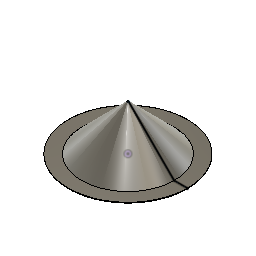
stage assembly v116 (Autodesk Fusion 360 archive; units mm, degrees)
design "electrode v2"
Autodesk Fusion 360 part; units mm, degrees
sketch "Sketch1" plane through (0, 0, 0) normal (0, 0, 1) x (1, 0, 0)
  line L0 (0.0652, 3.4348) -> (3.5, 0)
  line L1 (3.5, 0) -> (4.5, 0)
  line L2 (0.0298, 3.3994) -> (3.4793, -0.05)
  line L3 (3.4793, -0.05) -> (4.5, -0.05)
  line L4 (0.0652, 3.4348) -> (0.0298, 3.3994)
  line L5 (4.5, -0.05) -> (4.5, 0)
  dimension "d1" = 3.5
  dimension "d2" = 1
  dimension "d3" = 45
  dimension "d4" = 0.05
  constraint horizontal L1
  constraint horizontal origin L0.end
  constraint perpendicular L1 L5
  measures "d1" distance of origin L0.end
  measures "d2" distance of L0.end L1.end
  measures "d3" angle of L0 L1
revolve "Revolve1" add sketch "Sketch1" angle 360 about axis through (0, 1.75, 0) along (0, 1, 0)

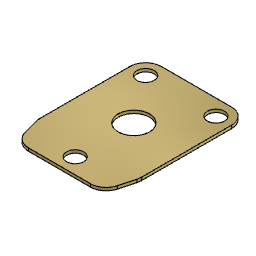
design "smb electrode top ground"
Autodesk Fusion 360 part; units mm, degrees
sketch "Sketch1" plane through (0, 0, 0) normal (0, 1, 0) x (1, 0, 0)
  circle A0 centre (-4.5, 13.5) radius 1.1
  circle A1 centre (4.5, 13.5) radius 1.1
  line L0 (0, -20) -> (0, -2.5) construction
  circle A2 centre (0, 0) radius 1.1
  circle A3 centre (0, 7.5) radius 2
  line L1 (-6.5, -2) -> (6.5, -2)
  line L2 (6.5, -2) -> (6.5, 15.5)
  line L3 (-6.5, -2) -> (-6.5, 15.5)
  line L4 (6.5, 15.5) -> (-6.5, 15.5)
  line L5 (-5.5, -2) -> (-6.5, 1.7321)
  line L6 (5.5, -2) -> (6.5, 1.7321)
  dimension "d1" = 2.2
  dimension "d2" = 2.2
  dimension "d3" = 9
  dimension "d4" = 13.5
  dimension "d5" = 2.2
  dimension "d6" = 7.5
  dimension "d7" = 4
  dimension "d8" = 13
  dimension "d9" = 2
  dimension "d10" = 2
  dimension "d15" = 30
  dimension "d16" = 11
  constraint horizontal A0.centre A1.centre
  constraint symmetric A0.centre A1.centre L0
  constraint coincident A2.centre origin
  constraint vertical A2.centre A3.centre
  constraint horizontal L1
  constraint perpendicular L1 L2
  constraint perpendicular L1 L3
  constraint perpendicular L2 L4
  constraint coincident L1 L5.start
  constraint coincident L3 L5.end
  constraint coincident L1 L6.start
  constraint coincident L2 L6.end
  constraint symmetric L0 L5 L6
  measures "d1" diameter of A0
  measures "d2" diameter of A1
  measures "d3" horizontal distance of A0.centre A1.centre
  measures "d4" vertical distance of A2.centre A1.centre
  measures "d5" diameter of A2
  measures "d6" distance of A2.centre A3.centre
  measures "d7" diameter of A3
  measures "d8" distance of L1.start L1.end
  measures "d9" distance of A2.centre L1
  measures "d10" distance of A1.centre L4
  measures "d15" angle of L5 L6
  measures "d16" distance of L5.start L6.start
extrude "Extrude1" add sketch "Sketch1" along normal blind 0.38 contours L1 L2 L3 L4 L5 L6
fillet "Fillet1" radius 2 6 edges at (-6.5, 0.19, -15.5) (6.5, 0.19, -15.5) (-5.5, 0.19, 2) (-6.5, 0.19, -1.7321) (5.5, 0.19, 2) (6.5, 0.19, -1.7321)

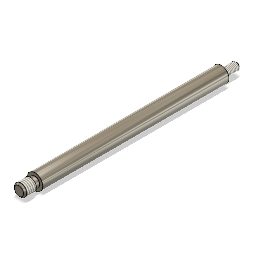
design "stage standoffs"
Autodesk Fusion 360 part; units mm, degrees
sketch "Sketch1" plane through (0, 0, 0) normal (1, 0, 0) x (0, 0, -1)
  line L0 (0, 0) -> (-137, 0)
  line L1 (-137, 0) -> (-137, 4)
  line L2 (-137, 4) -> (-127, 4)
  line L3 (-127, 4) -> (-127, 5)
  line L4 (-127, 5) -> (-10, 5)
  line L5 (-10, 5) -> (-10, 2.5)
  line L6 (-10, 2.5) -> (0, 2.5)
  line L7 (0, 2.5) -> (0, 0)
  line L8 (-127, 4) -> (-127, 3)
  line L9 (-127, 3) -> (-130, 3)
  line L10 (-130, 3) -> (-130, 4)
  dimension "d1" = 117
  dimension "d2" = 4
  dimension "d3" = 10
  dimension "d4" = 10
  dimension "d5" = 2.5
  dimension "d6" = 5
  dimension "d7" = 3
  dimension "d8" = 1
  measures "d2" distance of L0 L2
  measures "d3" distance of L1 L3
  measures "d5" distance of L0 L6
  measures "d6" distance of L0 L4
  measures "d8" distance of L2 L9
revolve "Revolve1" add sketch "Sketch1" angle 360 about axis through (0, 0, 0) along (0, 0, 1) contours L0 L1 L2 L3 L4 L5 L6 L7 L8 L9 L10
thread "Thread1" "ISO Metric profile 8.0 M8x1.25 6g" major diameter 7.866 minor diameter 6.4455 pitch 1.25 angle 60 resizes the face on face at (0.3983, 3.9801, 132.3333)
thread "Thread2" "ISO Metric profile 5.0 M5x0.8 6g" major diameter 4.901 minor diameter 3.9895 pitch 0.8 angle 60 resizes the face on face at (-0.2489, 2.4876, 6.6667)
chamfer "Chamfer1" distance 1 angle 45 2 edges at (-1.4222, -3.6668, 137) (-0.8861, -2.2847, 0)

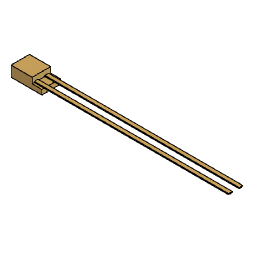
design "Lakeshore DT 670 SD Omega CY 670 SD"
Autodesk Fusion 360 part; units mm, degrees
sketch "Sketch1" plane through (0, 0, 0) normal (0, 0, 1) x (1, 0, 0)
  line L0 (0, 0) -> (3.175, 0)
  line L1 (3.175, 0) -> (3.175, 0.5)
  line L2 (3.175, 0.5) -> (2.175, 0.5)
  line L3 (2.175, 0.5) -> (2.175, 1.08)
  line L4 (2.175, 1.08) -> (0, 1.08)
  line L5 (0, 1.08) -> (0, 0)
  dimension "d1" = 1.08
  dimension "d2" = 3.175
  dimension "d3" = 1
  dimension "d4" = 0.5
  constraint coincident L0.start L5.end
  constraint horizontal L0
  constraint perpendicular L0 L1
  constraint perpendicular L1 L2
  constraint perpendicular L0 L3
  constraint perpendicular L3 L4
  constraint perpendicular L0 L5
  measures "d1" distance of L4.end L0.start
  measures "d2" distance of L0.start L0.end
  measures "d3" distance of L1.end L2.end
  measures "d4" distance of L0.end L1.end
extrude "Extrude1" add sketch "Sketch1" along normal blind 1.905
sketch "Sketch2" plane through (0, 0.5, 0) normal (0, 1, 0) x (-1, 0, 0)
  line L0 (-3.175, 0) -> (-2.175, 0)
  line L1 (-2.175, 0) -> (-2.175, 1.905)
  line L2 (-2.175, 1.905) -> (-3.175, 1.905)
  line L3 (-3.175, 1.905) -> (-3.175, 0)
  line L4 (-2.175, 0.2225) -> (-22.175, 0.2225)
  line L5 (-22.175, 0.2225) -> (-22.175, 0.6035)
  line L6 (-22.175, 0.6035) -> (-2.175, 0.6035)
  line L7 (-2.175, 0.6035) -> (-2.175, 0.2225)
  line L8 (-3.175, 0.9525) -> (0, 0.9525) construction
  line L9 (-2.175, 1.6825) -> (-22.175, 1.6825)
  line L10 (-22.175, 1.3015) -> (-2.175, 1.3015)
  line L11 (-22.175, 1.6825) -> (-22.175, 1.3015)
  line L12 (-2.175, 1.3015) -> (-2.175, 1.6825)
  dimension "d7" = 0.381
  dimension "d8" = 19
  dimension "d9" = 0.698
  constraint horizontal L4
  constraint vertical L5
  constraint horizontal L6
  constraint vertical L7
  constraint collinear L1 L7
  constraint midpoint L3 L8.start
  constraint perpendicular L3 L8
  constraint symmetric L4.start L8 L9.start
  constraint symmetric L4.end L8 L9.end
  constraint symmetric L5.end L8 L10.start
  constraint symmetric L6.end L8 L10.end
  measures "d7" distance of L4.end L5.end
  measures "d8" distance of L3 L5
  measures "d9" distance of L6 L10
extrude "Extrude2" add sketch "Sketch2" along normal blind 0.102 contours L3 L4 L5 L6 | L1 L3 L4 L6 L7 | L3 L9 L10 L11 | L1 L3 L9 L10 L12

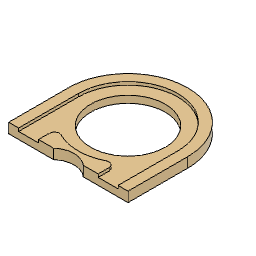
design "smb electrode insulators"
Autodesk Fusion 360 part; units mm, degrees
sketch "Sketch1" plane through (0, 0, 0) normal (0, 1, 0) x (1, 0, 0)
  line L0 (0, 0) -> (12, 0)
  line L1 (12, 0) -> (12, -12)
  line L2 (12, -12) -> (0, -12)
  line L3 (0, -12) -> (0, 0)
  circle A0 centre (6, -6) radius 3.75
  line L4 (6, 0) -> (6, -12) construction
  circle A1 centre (6, -6) radius 5
  line L5 (2, -12) -> (2, -9) construction
  line L6 (1, -12) -> (1, -6)
  line L7 (3, -10) -> (3, -12)
  arc A2 (7.5, -12) -> (4.5, -12) centre (6, -13.7) ccw
  dimension "d1" = 12
  dimension "d2" = 12
  dimension "d3" = 7.5
  dimension "d4" = 10
  dimension "d5" = 4
  dimension "d6" = 2
  dimension "d16" = 3
  dimension "d17" = 1.7
  constraint horizontal L0
  constraint vertical L1
  constraint horizontal L2
  constraint vertical L3
  constraint coincident L0.start L3.end
  constraint midpoint L0 L4.start
  constraint midpoint L2 L4.end
  constraint midpoint A0.centre L4
  constraint concentric A0 A1
  constraint coincident L2 L5.start
  constraint perpendicular L2 L5
  constraint coincident L2 L6.start
  constraint coincident A1 L6.end
  constraint perpendicular L2 L6
  constraint coincident A1 L7.start
  constraint coincident L2 L7.end
  constraint perpendicular L2 L7
  constraint coincident A1 L5.end
  constraint coincident L2 A2.start
  constraint coincident L2 A2.end
  constraint coincident L4 A2.centre
  measures "d1" distance of L0.start L2.end
  measures "d2" distance of L1.end L2.end
  measures "d3" diameter of A0
  measures "d4" diameter of A1
  measures "d5" distance of L4.end L5
  measures "d6" distance of L6 L7
  measures "d16" distance of A2.end A2.start
  measures "d17" distance of L2 A2.centre
extrude "Extrude1" add sketch "Sketch1" against normal blind 1 contours L0 L1 L2 L3 A1 L6 L7 A2 | L2 A1 L6 L7 | A1
extrude "Extrude2" cut sketch "Sketch1" against normal blind 0.3 contours A1
extrude "Extrude3" cut sketch "Sketch1" against normal blind 0.3 contours L2 A1 L6 L7
ref_plane "WorkPlane1" through (6, -0.5, 6) normal (1, 0, 0) x (0, 0, 1)
mirror "Mirror1" about plane through (6, -0.5, 6) normal (1, 0, 0) of "Extrude3"
fillet "Fillet1" radius 6 2 edges at (0, -0.5, 0) (12, -0.5, 0)
fillet "Fillet2" radius 0.5 2 edges at (3, -0.15, 10) (9, -0.15, 10)
equation "d3 = ( 3.75 * 2 ) * 1 mm"

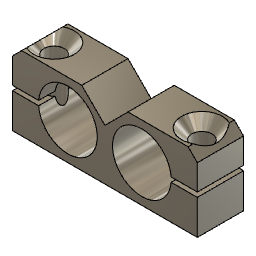
design "SMB plug holder"
Autodesk Fusion 360 part; units mm, degrees
sketch "Sketch1" plane through (0, 0, 0) normal (0, 0, 1) x (1, 0, 0)
  line L0 (0, 0) -> (20, 0)
  line L1 (20, 0) -> (20, 8)
  line L2 (20, 8) -> (0, 8)
  line L3 (0, 8) -> (0, 0)
  circle A0 centre (6, 4) radius 3.175
  circle A1 centre (14, 4) radius 3.175
  line L4 (10, 0) -> (10, 8) construction
  line L5 (7.5, 8) -> (10, 5.5)
  line L6 (10, 5.5) -> (12.5, 8)
  dimension "d1" = 6.35
  dimension "d2" = 6.35
  dimension "d3" = 8
  dimension "d4" = 4
  dimension "d5" = 20
  dimension "d6" = 8
  dimension "d9" = 2.5
  constraint horizontal L0
  constraint vertical L1
  constraint horizontal L2
  constraint vertical L3
  constraint coincident L0.start L3.end
  constraint horizontal A0.centre A1.centre
  constraint midpoint L0 L4.start
  constraint midpoint L2 L4.end
  constraint symmetric A0.centre A1.centre L4
  constraint coincident L2 L5.start
  constraint coincident L4 L5.end
  constraint coincident L2 L6.end
  constraint perpendicular L5 L6
  constraint symmetric L4 L5 L6
  measures "d1" diameter of A0
  measures "d2" diameter of A1
  measures "d3" distance of A0.centre A1.centre
  measures "d4" distance of L0 A0.centre
  measures "d5" distance of L0.start L0.end
  measures "d6" distance of L0 L2
  measures "d9" distance of L2 L5.end
extrude "Extrude1" add sketch "Sketch1" against normal blind 5 contours L0 L1 L2 L3 L5 L6
sketch "Sketch2" plane through (0, 8, 0) normal (0, 1, 0) x (-1, 0, 0)
  line L0 (-12.5, 0) -> (-20, 0)
  line L1 (-20, 0) -> (-20, -5)
  line L2 (-20, -5) -> (-12.5, -5)
  line L3 (-12.5, -5) -> (-12.5, 0)
  line L4 (0, 0) -> (0, -5)
  line L5 (-20, 0) -> (-20, -5)
  line L6 (-20, -2.5) -> (0, -2.5) construction
  line L7 (-10, 0) -> (-10, -5)
  point P0 (-2, -2.5)
  point P1 (-18, -2.5)
  dimension "d10" = 2
  dimension "d19" = 16
  constraint midpoint L1 L6.start
  constraint midpoint L4 L6.end
  constraint coincident L6 P0
  constraint coincident L6 P1
  constraint symmetric P0 P1 L7
  measures "d10" distance of L4 P0
  measures "d19" distance of P0 P1
chamfer "Chamfer1" distance 1 angle 45 2 edges at (20, 8, -2.5) (0, 8, -2.5)
hole "Hole1" at (2, 8, -2.5) at (18, 8, -2.5) direction (0, -1, 0) diameter 2.2 depth 10 tip angle 118 countersink diameter 4.4 countersink angle 90
ref_plane "WorkPlane1" through (16.25, 4, -2.5) normal (0, 1, 0) x (1, 0, 0)
sketch "Sketch3" plane through (16.25, 4, -3.5) normal (0, 1, 0) x (1, 0, 0)
  line L0 (0, 6) -> (6.8751, 6)
  line L1 (6.8751, 6) -> (6.8751, -6.5674)
  line L2 (6.8751, -6.5674) -> (0, -6.5674)
  line L3 (0, -6.5674) -> (0, 6)
  line L4 (-17, 6) -> (-11.0861, 6)
  line L5 (-11.0861, 6) -> (-11.0861, -6.5674)
  line L6 (-11.0861, -6.5674) -> (-17, -6.5674)
  line L7 (-17, -6.5674) -> (-17, 6)
  constraint horizontal L0
  constraint vertical L1
  constraint horizontal L2
  constraint vertical L3
  constraint horizontal L4
  constraint vertical L5
  constraint horizontal L6
  constraint vertical L7
extrude "Extrude2" cut sketch "Sketch3" along normal mid plane 0.5

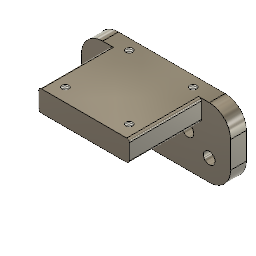
design "EX-0009723-000-XYZ-SLC-1730 z connector"
Autodesk Fusion 360 part; units mm, degrees
sketch "Sketch2" plane through (0, 0, 0) normal (0, 0, 1) x (1, 0, 0)
  arc A0 (18.5, 20) -> (18, 20.5) centre (18, 20) ccw
  line L0 (18.5, 20) -> (18.5, 8.6168)
  arc A1 (18.5, 8.6168) -> (21.6842, 3.6281) centre (24, 8.6168) ccw
  arc A2 (20, -4) -> (21.6842, 3.6281) centre (20, 0) ccw
  line L1 (20, -4) -> (0, -4)
  arc A3 (-1.6842, 3.6281) -> (0, -4) centre (0, 0) ccw
  arc A4 (-1.6842, 3.6281) -> (1.5, 8.6168) centre (-4, 8.6168) ccw
  line L2 (1.5, 8.6168) -> (1.5, 20)
  arc A5 (2, 20.5) -> (1.5, 20) centre (2, 20) ccw
  line L3 (2, 20.5) -> (18, 20.5)
  circle A6 centre (20, 0) radius 1.1
  circle A7 centre (0, 0) radius 1.1
  line L4 (24, 9) -> (-4, 9)
  line L5 (-4, 0) -> (-4, 9)
  line L6 (24, 0) -> (24, 9)
  line L7 (1.5, 9) -> (1.5, 5)
  line L8 (1.5, 5) -> (18.5, 5)
  line L9 (18.5, 5) -> (18.5, 9)
  line L10 (10, -4) -> (10, 20.5) construction
  point P0 (4, 2.5)
  point P1 (16, 2.5)
  dimension "d2" = 9
  dimension "d6" = 4
  dimension "d20" = 12
  dimension "d21" = 2.5
  constraint horizontal L4
  constraint coincident A3 L5.start
  constraint coincident A2 L6.start
  constraint tangent A2 L6
  constraint tangent A3 L5
  constraint vertical L6
  constraint vertical L5
  constraint coincident L4 L7.start
  constraint coincident L2 L7.start
  constraint perpendicular L4 L7
  constraint perpendicular L0 L8
  constraint coincident L4 L9.end
  constraint coincident L0 L9.end
  constraint perpendicular L4 L9
  constraint midpoint L1 L10.start
  constraint midpoint L3 L10.end
  constraint horizontal P0 P1
  constraint symmetric L10 P0 P1
  measures "d2" distance of A3.centre L4
  measures "d6" distance of L4 L8
  measures "d20" distance of P0 P1
  measures "d21" distance of L8 P1
ref_plane "WorkPlane1" through (0, 9, 0) normal (0, 1, 0) x (0, 0, 1)
sketch "Sketch3" plane through (0, 9, 0) normal (0, 1, 0) x (1, 0, 0)
  circle A0 centre (4, -13.5) radius 0.625
  circle A1 centre (4, -13.5) radius 0.625
  circle A2 centre (16, -13.5) radius 0.625
  circle A3 centre (16, -13.5) radius 0.625
  circle A4 centre (16, -1.5) radius 0.625
  circle A5 centre (16, -1.5) radius 0.625
  circle A6 centre (4, -1.5) radius 0.625
  circle A7 centre (4, -1.5) radius 0.625
  dimension "d4" = 12
  dimension "d5" = 12
  measures "d4" distance of A2.centre A4.centre
  measures "d5" distance of A0.centre A2.centre
extrude "Extrude1" add sketch "Sketch2" along normal blind 2.5 and the other way blind 0.5 contours L0 A1 A2 L4 L6 L9 | L0 L2 L4 L7 L8 L9 | A1 A2 L1 A3 A4 L7 L8 L9 | A3 A4 L2 L4 L5 L7
extrude "Extrude2" add sketch "Sketch2" along normal blind 16 contours L0 L2 L4 L7 L8 L9
hole "Hole1" at (4, 9, 13.5) at (16, 9, 13.5) at (16, 9, 1.5) at (4, 9, 1.5) direction (0, -1, 0) diameter 1.271 depth 6.5 tip angle 118
thread "Thread1" "ISO Metric profile 1.6 M1.6x0.35 6H"
fillet "Fillet1" radius 4 2 edges at (24, 9, 1) (-4, 9, 1)
fillet "Fillet1" radius 0.5 4 edges at (18.5, 9, 9.25) (1.5, 9, 9.25) (18.5, 5, 9.25) (1.5, 5, 9.25)
hole "Hole2" at (16, 2.5, 0) at (4, 2.5, 0) direction (0, 0, 1) diameter 2.2 depth 11 tip angle 118
hole "Hole3" at (16, 2.5, 0) at (4, 2.5, 0) direction (0, 0, -1) diameter 2.2 depth 11 tip angle 118

design "base plate"
Autodesk Fusion 360 part; units mm, degrees
sketch "Sketch1" plane through (0, 0, 0) normal (0, 1, 0) x (1, 0, 0)
  circle A0 centre (0, 0) radius 20
  line L0 (1.75, 0) -> (22.5, 0) construction
  line L1 (0, -20) -> (0, -2.5) construction
  line L2 (-35, 91) -> (35, 91)
  line L3 (35, 91) -> (35, -35)
  line L4 (35, -35) -> (-35, -35)
  line L5 (-35, -35) -> (-35, 91)
  line L6 (-8.55, 91) -> (-8.55, 25)
  line L7 (-8.55, 25) -> (8.55, 25)
  line L8 (8.55, 25) -> (8.55, 91)
  line L9 (-12.5, -25) -> (12.5, -25) construction
  circle A1 centre (-12.5, -25) radius 5
  circle A2 centre (12.5, -25) radius 5
  line L10 (-7.7, 86) -> (-7.7, 35)
  arc A3 (-7.7, 35) -> (-5.7, 35) centre (-6.7, 35) ccw
  line L11 (-5.7, 35) -> (-5.7, 86)
  arc A4 (-5.7, 86) -> (-7.7, 86) centre (-6.7, 86) ccw
  line L12 (-6.7, 86) -> (-6.7, 35) construction
  line L13 (-33, 91) -> (-33, 41)
  arc A5 (-33, 41) -> (-23, 41) centre (-28, 41) ccw
  line L14 (-23, 41) -> (-23, 91)
  line L15 (-33, 10) -> (-33, -10)
  arc A6 (-33, -10) -> (-20.592, -7.744) centre (-26.5909, -10) ccw
  arc A7 (-20.592, 7.744) -> (-33, 10) centre (-26.5909, 10) ccw
  line L16 (-26.5909, 10) -> (-26.5909, -10) construction
  line L17 (-25, -25) -> (-25, 25) construction
  line L18 (-25, 0) -> (-26.5909, 0) construction
  arc A8 (-20.592, 7.744) -> (-20.592, -7.744) centre (0, 0) ccw
  point P0 (25, 0)
  point P1 (0, -25)
  point P2 (-6.7, 66)
  point P3 (-6.7, 40)
  point P4 (6.7, 40)
  point P5 (6.7, 66)
  point P6 (-12.5, -25)
  point P7 (12.5, -25)
  point P8 (-25, 25)
  point P9 (25, 25)
  point P10 (25, -25)
  point P11 (-25, -25)
  dimension "d1" = 40
  dimension "d4" = 26
  dimension "d5" = 13.4
  dimension "d6" = 40
  dimension "d7" = 70
  dimension "d8" = 35
  dimension "d10" = 17.1
  dimension "d14" = 25
  dimension "d15" = 25
  dimension "d28" = 10
  dimension "d29" = 10
  dimension "d32" = 50
  dimension "d33" = 50
  dimension "d63" = 2
  dimension "d64" = 5
  dimension "d65" = 10
  dimension "d66" = 20
  dimension "d67" = 5
  dimension "d71" = 2
  dimension "d72" = 10
  dimension "d73" = 50
  dimension "d79" = 20
  dimension "d80" = 2
  constraint coincident A0.centre A8.centre
  constraint coincident P0 L0
  constraint horizontal P3 P4
  constraint vertical P4 P5
  constraint horizontal P2 P5
  constraint vertical P2 P3
  constraint symmetric L1 P3 P4
  constraint horizontal L2
  constraint vertical L3
  constraint horizontal L4
  constraint vertical L5
  constraint symmetric L1 L3 L5
  constraint coincident L2 L6.start
  constraint perpendicular L2 L6
  constraint perpendicular L6 L7
  constraint coincident L2 L8.end
  constraint perpendicular L2 L8
  constraint coincident L9 P6
  constraint coincident L9 P7
  constraint symmetric L1 P6 P7
  constraint coincident P7 L9.end
  constraint coincident P6 L9.start
  constraint horizontal P10 P11
  constraint vertical P8 P11
  constraint horizontal P8 P9
  constraint vertical P9 P10
  constraint symmetric L0 P9 P10
  constraint symmetric L1 P10 P11
  constraint tangent L10 A3
  constraint tangent A3 L11
  constraint parallel L10 L11
  constraint tangent L11 A4
  constraint tangent L10 A4
  constraint parallel L6 L12
  constraint coincident P3 L12
  constraint coincident L2 L13.start
  constraint perpendicular L2 L13
  constraint tangent L13 A5
  constraint coincident L2 L14.end
  constraint perpendicular L2 L14
  constraint tangent A5 L14
  constraint tangent L15 A6
  constraint tangent L15 A7
  constraint vertical L16
  constraint coincident P11 L17.start
  constraint coincident P8 L17.end
  constraint midpoint L17 L18.start
  constraint midpoint L16 L18.end
  constraint horizontal L18
  constraint collinear L13 L15
  constraint tangent A6 A8
  measures "d1" diameter of A0
  measures "d4" vertical distance of P4 P5
  measures "d5" horizontal distance of P2 P5
  measures "d6" distance of L0 P4
  measures "d7" distance of L3 L5
  measures "d8" distance of L0 L4
  measures "d10" distance of L6 L8
  measures "d14" distance of L0 L9
  measures "d15" distance of P6 P7
  measures "d28" diameter of A1
  measures "d29" diameter of A2
  measures "d32" distance of P8 P11
  measures "d33" distance of P10 P11
  measures "d63" diameter of A3
  measures "d64" distance of P3 A3.centre
  measures "d65" distance of L7 A3.centre
  measures "d66" distance of P2 A4.centre
  measures "d67" distance of L2 A4.centre
  measures "d71" distance of L5 L13
  measures "d72" distance of L13 L14
  measures "d73" distance of L2 A5.centre
  measures "d79" distance of A7.centre A6.centre
  measures "d80" distance of A0 A8
extrude "Extrude1" add sketch "Sketch1" along normal blind 4 contours L2 L3 L4 L5 L6 L7 L8 L13 A5 L14 | L2 L13 A5 L14 | L2 L6 L7 L8 | A1 | A2 | L10 A3 L11 A4 | L15 A6 A7 A8 makes body 1
extrude "Extrude7" cut sketch "Sketch1" along normal through all contours L10 A3 L11 A4 bodies 1
mirror "Mirror1" about plane through (0, 0, 0) normal (1, 0, 0) of "Extrude7"
extrude "Extrude2" cut sketch "Sketch1" along normal blind 0.5 contours L2 L6 L7 L8 | A1 | A2 | L10 A3 L11 A4 bodies 1
hole "Hole1" at (0, 0, 25) at (-12.5, 0, 25) at (12.5, 0, 25) direction (0, 1, 0) diameter 4 end through all bodies 1
hole "Hole3" at (-25, 0, 25) at (25, 0, 25) at (-25, 0, -25) at (25, 0, -25) direction (0, 1, 0) diameter 9 end through all bodies 1
extrude "Extrude8" cut sketch "Sketch1" along normal blind 1.5 contours L2 L13 A5 L14 | L15 A6 A7 A8 bodies 1
mirror "Mirror2" about plane through (0, 0, 0) normal (1, 0, 0) of "Extrude8"
ref_plane "WorkPlane1" through (0, 2, -28) normal (0, -1, 0) x (-1, 0, 0)
mirror "Mirror3" about plane through (0, 2, -28) normal (0, -1, 0) of "Extrude8", "Mirror2"
sketch "Sketch2" plane through (0, 0, 0) normal (0, 1, 0) x (1, 0, 0)
  line L0 (35, -35) -> (-35, -35)
  line L1 (-35, -35) -> (-35, 91)
  line L2 (35, 91) -> (35, -35)
  line L3 (-35, 35) -> (35, 35)
  circle A0 centre (-25, -25) radius 4.5
  circle A1 centre (25, -25) radius 4.5
  circle A2 centre (25, 25) radius 4.5
  circle A3 centre (-25, 25) radius 4.5
  circle A4 centre (-25, -25) radius 6.25
  circle A5 centre (0, 0) radius 20
  line L4 (1.75, 0) -> (22.5, 0)
  line L5 (0, -20) -> (0, -2.5)
  point P0 (-30, -5)
  point P1 (30, -5)
  point P2 (0, 30)
  dimension "d38" = 70
  dimension "d39" = 12.5
  dimension "d40" = 60
  dimension "d41" = 30
  dimension "d42" = 5
  constraint coincident L2 L3.end
  constraint perpendicular L2 L3
  constraint concentric A0 A4
  constraint horizontal P0 P1
  constraint symmetric P0 P1 L5
  measures "d38" distance of L0 L3
  measures "d39" diameter of A4
  measures "d40" horizontal distance of P0 P1
  measures "d41" distance of P2 L4
  measures "d42" distance of P1 L4
extrude "Extrude3" add sketch "Sketch2" along normal blind 4 from surface at 15 separate body contours L0 L1 L2 L3 | A4 makes body 2
hole "Hole4" at (-30, 0, 5) at (30, 0, 5) at (0, 0, -30) direction (0, 1, 0) diameter 5.3 end through all bodies 2
fillet "Fillet2" radius 5 8 edges at (35, 2, 35) (-35, 2, 35) (-35, 2, -91) (35, 2, -91) (35, 17, 35) (35, 17, -35) (-35, 17, 35) (-35, 17, -35) on bodies 1 2
extrude "Extrude4" add sketch "Sketch2" along normal up to surface (29 mm away) from surface at -5 separate body contours A0 makes body 3
extrude "Extrude5" add sketch "Sketch2" along normal up to surface (11 mm away) from surface at 4 contours A4 bodies 3
hole "Hole5" at (-25, -5, 25) direction (0, 1, 0) diameter 5.5 end through all bodies 3
extrude "Extrude6" add sketch "Sketch2" against normal blind 6 separate body contours A4 makes body 4
fillet "Fillet3" radius 4 2 edges at (-8.55, 0.25, -25) (8.55, 0.25, -25) on bodies 1
fillet "Fillet4" radius 1 28 edges at (25.4444, 2.5, -16.3057) (33, 2.5, 0) (25.4444, 2.5, 16.3057) (22, 2.5, 0) (33, 2.5, -65.5) (28, 2.5, -36) (23, 2.5, -66) (-22, 2.5, 0) (-25.4444, 2.5, -16.3057) (-33, 2.5, 0) (-25.4444, 2.5, 16.3057) (-33, 2.5, -65.5) (-28, 2.5, -36) (-23, 2.5, -66) (33, 1.5, -65.5) (28, 1.5, -36) (23, 1.5, -66) (22, 1.5, 0) (25.4444, 1.5, -16.3057) (33, 1.5, 0) (25.4444, 1.5, 16.3057) (-33, 1.5, -65.5) (-28, 1.5, -36) (-23, 1.5, -66) (-33, 1.5, 0) (-25.4444, 1.5, 16.3057) (-22, 1.5, 0) (-25.4444, 1.5, -16.3057) on bodies 1
sketch "Sketch3" plane through (0, 0, 0) normal (0, 0, 1) x (1, 0, 0)
  line L0 (30, 0) -> (-30, 0)
  line L1 (-30, 4) -> (30, 4)
  point P0 (-25, 9.5)
  point P1 (-25, -2)
  dimension "d82" = 2
  dimension "d83" = 5.5
  measures "d82" distance of P1 L0
  measures "d83" distance of P0 L1
hole "Hole6" at (-25, 9.5, 0) direction (0, 0, 1) diameter 5 end through all bodies 3
move_face "OffsetFaces1" offset -0.05 2 faces at (-20.5224, 18, 25.4481) (-20.5224, -2, 25.4481) on bodies 3
chamfer "Chamfer1" distance 0.25 angle 45 4 edges at (-29.45, 24, 25) (-25.9944, 24, 27.5639) (-24.0056, -5, 27.5639) (-29.45, -5, 25) on bodies 3
move_face "OffsetFaces2" offset -0.05 1 faces at (-20.5056, -4, 25.2243) on bodies 4
sketch "Sketch4" plane through (0, 0, 0) normal (0, 1, 0) x (-1, 0, 0)
  circle A0 centre (25, 25) radius 4.55
  circle A1 centre (25, 25) radius 6.25
  circle A2 centre (25, 21.6) radius 1.55
  dimension "d88" = 3.1
  dimension "d89" = 3.4
  constraint vertical A0.centre A2.centre
  measures "d88" diameter of A2
  measures "d89" distance of A0.centre A2.centre
extrude "Extrude9" cut sketch "Sketch4" against normal through all contours A0 A2 picked at (25.3493, 20.3519) bodies 4
pattern_circular "C-Pattern1" count 6 over 360 about axis through (-25, 0, 25) along (0, -1, 0) of "Extrude9"
chamfer "Chamfer2" distance 0.25 angle 45 2 edges at (-30.827, 0, 27.2601) (-30.827, -6, 22.7399) on bodies 4
copy_body "Body->Comp1" bodies 1 removing the originals makes body 5 in component "bottom plate"
copy_body "Body->Comp2" bodies 2 removing the originals makes body 6 in component "top plate"
copy_body "Body->Comp3" bodies 3 removing the originals makes body 7 in component "vespel seperator"
copy_body "Body->Comp4" bodies 4 removing the originals makes body 8 in component "vespel spacer"
component_pattern "component pattern"
component "bottom plate" placed x (1, 0, 0) y (0, 1, 0) z (0, 0, 1) at (0, 0, 0)
component "top plate" placed x (1, 0, 0) y (0, 1, 0) z (0, 0, 1) at (0, 0, 0)
component "vespel seperator" placed x (1, 0, 0) y (0, 1, 0) z (0, 0, 1) at (0, 0, 0)
component "vespel spacer" placed x (1, 0, 0) y (0, 1, 0) z (0, 0, 1) at (0, 0, 0)
component "vespel spacer" placed x (1, 0, 0) y (0, 1, 0) z (0, 0, 1) at (0, 26, 0)
component "vespel seperator" placed x (0, 0, -1) y (0, 1, 0) z (1, 0, 0) at (0, 0, 0)
component "vespel spacer" placed x (0, 0, -1) y (0, 1, 0) z (1, 0, 0) at (0, 0, 0)
component "vespel spacer" placed x (0, 0, -1) y (0, 1, 0) z (1, 0, 0) at (0, 26, 0)
component "vespel seperator" placed x (-1, 0, 0) y (0, 1, 0) z (0, 0, -1) at (0, 0, 0)
component "vespel spacer" placed x (-1, 0, 0) y (0, 1, 0) z (0, 0, -1) at (0, 0, 0)
component "vespel spacer" placed x (-1, 0, 0) y (0, 1, 0) z (0, 0, -1) at (0, 26, 0)
component "vespel seperator" placed x (0, 0, 1) y (0, 1, 0) z (-1, 0, 0) at (0, 0, 0)
component "vespel spacer" placed x (0, 0, 1) y (0, 1, 0) z (-1, 0, 0) at (0, 0, 0)
component "vespel spacer" placed x (0, 0, 1) y (0, 1, 0) z (-1, 0, 0) at (0, 26, 0)

design "Lakeshore CO clamp"
Autodesk Fusion 360 part; units mm, degrees
sketch "Sketch1" plane through (0, 0, 0) normal (0, 0, 1) x (1, 0, 0)
  line L0 (0, 0) -> (0, 3.2)
  line L1 (0, 3.2) -> (-7.9, 3.2)
  line L2 (-7.9, 3.2) -> (-7.9, 0.9)
  line L3 (-7.9, 0.9) -> (-1, 0.9)
  line L4 (-1, 0.9) -> (-1, 0)
  line L5 (-1, 0) -> (0, 0)
  dimension "d1" = 3.2
  dimension "d2" = 7.9
  dimension "d3" = 0.9
  dimension "d4" = 1
  constraint coincident L0.start L5.end
  constraint vertical L0
  constraint perpendicular L0 L1
  constraint perpendicular L1 L2
  constraint perpendicular L2 L3
  constraint perpendicular L1 L4
  constraint perpendicular L0 L5
  measures "d1" distance of L0.start L0.end
  measures "d2" distance of L0.end L1.end
  measures "d3" distance of L3.end L4.end
  measures "d4" distance of L4.end L0.start
extrude "Extrude1" add sketch "Sketch1" along normal blind 5.1
hole "Hole1" at (-3.95, 3.2, 2.55) direction (0, -1, 0) diameter 3.264 depth 5 tip angle 118
sketch "Sketch2" plane through (0, 0, 0) normal (0, 1, 0) x (1, 0, 0)
  circle A0 centre (-3.95, -2.55) radius 2
  circle A1 centre (-3.95, -2.55) radius 1.632
  dimension "d10" = 4
  constraint concentric A0 A1
  measures "d10" diameter of A0
extrude "Extrude2" add sketch "Sketch2" along normal up to surface (10.1 mm away) contours A1
